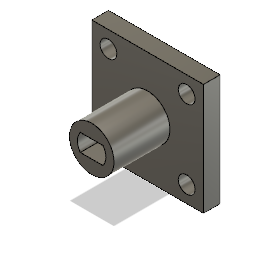
Fixateur roue (Autodesk Fusion 360 design; units mm, degrees)
Autodesk Fusion 360 part; units mm, degrees
sketch "Sketch1" plane through (0, 0, 0) normal (0, 0, 1) x (1, 0, 0)
  line L0 (2.55, 1.55) -> (-2.55, -1.55) construction
  line L1 (2.55, 1.55) -> (-2.55, -1.55) construction
  line L2 (-2.55, 1.55) -> (-2.55, -1.55)
  circle A0 centre (0, 0) radius 4
  line L3 (-2.55, 1.55) -> (2.55, -1.55) construction
  line L4 (-2.55, -1.55) -> (2.55, -1.55)
  line L5 (2.55, 1.55) -> (-2.55, 1.55)
  line L6 (2.55, 1.55) -> (-2.55, -1.55) construction
  line L7 (-2.55, 1.55) -> (2.55, -1.55) construction
  line L8 (-2.55, 1.55) -> (2.55, -1.55) construction
  circle A1 centre (0, 0) radius 2.55
  line L9 (2.55, -1.55) -> (2.55, 1.55)
  line L10 (-10, 10) -> (10, 10)
  line L11 (10, 10) -> (10, -10)
  line L12 (10, -10) -> (-10, -10)
  line L13 (-10, -10) -> (-10, 10)
  circle A2 centre (-7, 7) radius 1.5
  line L14 (0, 10) -> (0, 7.5)
  circle A3 centre (7, 7) radius 1.5
  line L15 (-10, 0) -> (-8.5, 0)
  circle A4 centre (-7, -7) radius 1.5
  circle A5 centre (7, -7) radius 1.5
  dimension "d1" = 5.1
  dimension "d2" = 5.1
  dimension "d3" = 3.1
  dimension "d4" = 8
  dimension "d5" = 5.1
  dimension "d6" = 5.1
  dimension "d7" = 20
  dimension "d8" = 20
  dimension "d9" = 3
  constraint coincident A0.centre L6
  constraint coincident A0.centre L3
  constraint coincident A0.centre A1.centre
  constraint parallel L4 L5
  constraint horizontal L5
  constraint coincident A0.centre L0
  constraint coincident A0.centre L8
  constraint concentric A0 A1
  constraint coincident A0.centre L1
  constraint coincident A0.centre L7
  constraint parallel L2 L9
  constraint horizontal L10
  constraint vertical L11
  constraint horizontal L12
  constraint vertical L13
  constraint midpoint L10 L14.start
  constraint perpendicular L10 L14
  constraint symmetric A2 L14 A3
  constraint midpoint L13 L15.start
  constraint perpendicular L13 L15
  constraint symmetric A2 L15 A4
  constraint symmetric L14 A4 A5
  measures "d1" distance of L0.end L3.end
  measures "d2" distance of L0.end L3.end
  measures "d3" distance of L2.start L0.end
  measures "d4" diameter of A0
  measures "d5" diameter of A1
  measures "d6" distance of L0.end L3.end
  measures "d7" distance of L10.start L12.end
  measures "d8" distance of L10.start L10.end
  measures "d9" diameter of A2
extrude "Extrude1" add sketch "Sketch1" along normal blind 10 contours L2 L5 A1 | L2 L4 A1 | L5 A1 | L4 A1 | L5 A1 L9 | L4 A1 L9 | A0 makes body 1
extrude "Extrude2" add sketch "Sketch1" against normal blind 3 separate body contours L10 L11 L12 L13 makes body 2
extrude "Extrude3" add sketch "Sketch1" against normal blind 3 contours L2 L5 A1 | L2 L4 A1 | L4 L5 A1 | L5 A1 | L4 A1 | L5 A1 L9 | L4 A1 L9 | A0 bodies 1 2
sketch "Sketch2" plane through (0, -1.55, 0) normal (0, 1, 0) x (-1, 0, 0)
  line L0 (-2.0248, 0) -> (2.0248, 0)
  line L1 (2.0248, 0) -> (2.0248, 10)
  line L2 (2.0248, 10) -> (-2.0248, 10)
  line L3 (-2.0248, 10) -> (-2.0248, 0)
  circle A0 centre (0.0464, 5) radius 1.5
  dimension "d18" = 3
  measures "d18" diameter of A0
extrude "Extrude4" cut sketch "Sketch2" against normal blind 3 contours A0 bodies 1
